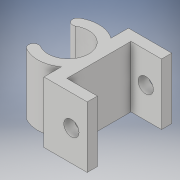
# Autodesk Inventor part: 6mm Weight Clamp
Saved by Autodesk Inventor 2019 (Build 230136000, 136)
## iProperties
Created: 2019-10-21
Part Number: 6mm Weight Clamp
Material: Generic
Document SubType Name: Modeling
Designer: 19879326
Density: 1 g/cm^3
Appearance: Default
Author: 19879326
Autodesk Inventor part; units mm, degrees
ref_plane "YZ Plane" through (0, 0, 0) normal (1, 0, 0) x (0, 1, 0)
ref_plane "XZ Plane" through (0, 0, 0) normal (0, 1, 0) x (-1, 0, 0)
ref_plane "XY Plane" through (0, 0, 0) normal (0, 0, 1) x (1, 0, 0)
sketch "Sketch1" plane through (0, 0, 0) normal (0, 1, 0) x (-1, 0, 0)
  line L0 (5.5, 8.3) -> (-3, 8.3)
  line L1 (-3, -8.3) -> (5.5, -8.3)
  line L2 (-3, 6.3) -> (3, 6.3)
  line L3 (3, 6.3) -> (3, -6.3)
  line L4 (3, -6.3) -> (-3, -6.3)
  arc A0 (11, 3.4641) -> (11, -3.4641) centre (9, 0) ccw
  line L5 (5.5, -8.3) -> (5.5, -4.8734)
  line L6 (5.5, 4.8734) -> (5.5, 8.3)
  line L7 (-3, 8.3) -> (-3, 6.3)
  line L8 (-3, -6.3) -> (-3, -8.3)
  arc A1 (11, 3.4641) -> (12, 5.1962) centre (11.5, 4.3301) ccw
  arc A2 (12, -5.1962) -> (11, -3.4641) centre (11.5, -4.3301) ccw
  arc A3 (5.5, -4.8734) -> (12, -5.1962) centre (9, 0) ccw
  arc A4 (12, 5.1962) -> (5.5, 4.8734) centre (9, 0) ccw
  point P0 (0, 0)
  point P1 (3, 0)
  point P2 (-6.8446, 0)
  point P3 (-6.8446, 0)
  point P4 (0, 6.3)
  point P5 (0, -6.3)
  dimension "d1" = 8
  dimension "d2" = 2.5
  dimension "d3" = 12.6
  dimension "d4" = 2
  dimension "d5" = 6
  dimension "d6" = 2.5
  dimension "d7" = 2.5
  dimension "d8" = 6
  dimension "d9" = 6
  dimension "d10" = 6
  constraints: 18 end point, 10 point on circle, 6 parallel, 5 centre point, 4 midpoint, 4 tangent, 3 perpendicular, 3 vertical alignment, 2 coincident, 2 collinear, 2 horizontal, 2 horizontal alignment
  measures "d1" diameter of A0
  measures "d2" horizontal distance of A3.centre A1.centre
  measures "d3" distance of L2.end L3.end
  measures "d4" distance of L4.end L1.start
  measures "d5" distance of point (3, 0) A0.centre
  measures "d6" distance between parallel lines of L3 L6
  measures "d7" distance between parallel lines of L3 L5
  measures "d8" radius of A4
  measures "d9" radius of A3
  measures "d10" distance of L2.start L2.end
extrude "Extrusion1" add sketch "Sketch1" along normal blind 12
sketch "Sketch2" plane through (-5.5, 0, 8.3) normal (0, 0, 1) x (1, 0, 0)
  circle A0 centre (5.4, 6) radius 1.5
  line L0 (2.5, 0) -> (2.5, 12) projected
  point P0 (5.5, 0)
  dimension "d13" = 2.9
  dimension "d14" = 6
  dimension "d15" = 3
  constraints: 1 centre point
  measures "d13" distance from line of L0 A0.centre
  measures "d14" vertical distance of point (5.5, 0) A0.centre
  measures "d15" diameter of A0
extrude "Extrusion2" cut sketch "Sketch2" against normal blind 65.75
body "Solid1"
